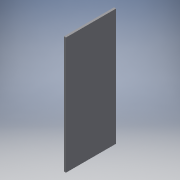
# Autodesk Inventor part: 15102898-16-P-0402
Saved by Autodesk Inventor 2017 (Build 210142000, 142)
## iProperties
Created: 2016-10-08
Part Number: 15102898-16-P-0402
Material: Aluminum 6061
Document SubType Name: Modeling
Designer: gus
Density: 2.7 g/cm^3
Appearance: Aluminum - Flat
Author: gus
Autodesk Inventor part; units mm, degrees
ref_plane "YZ Plane" through (0, 0, 0) normal (1, 0, 0) x (0, 1, 0)
ref_plane "XZ Plane" through (0, 0, 0) normal (0, 1, 0) x (-1, 0, 0)
ref_plane "XY Plane" through (0, 0, 0) normal (0, 0, 1) x (1, 0, 0)
sketch "Sketch1" plane through (0, 0, 0) normal (1, 0, 0) x (0, 1, 0)
  line L0 (0, 0) -> (177.8, 0)
  line L1 (177.8, 0) -> (177.8, -79.375)
  line L2 (177.8, -79.375) -> (0, -79.375)
  line L3 (0, -79.375) -> (0, 0)
  dimension "d0" = 177.8
  dimension "d1" = 79.375
  constraints: 8 end point, 2 parallel, 1 horizontal, 1 perpendicular
  measures "d0" distance of L1.end L2.end
  measures "d1" distance of L0.end L1.end
extrude "Extrusion1" add sketch "Sketch1" along normal blind 3.175
sketch "Sketch2" plane through (3.175, 0, 0) normal (1, 0, 0) x (0, 0, -1)
  line L0 (0, 177.8) -> (0, 0) projected
  line L1 (0, 0) -> (3.175, 0)
  line L2 (3.175, 0) -> (3.175, 177.8)
  line L3 (3.175, 177.8) -> (0, 177.8)
  line L4 (0, 177.8) -> (0, 0)
  dimension "d4" = 3.175
  constraints: 8 end point, 2 parallel, 1 horizontal, 1 perpendicular
  measures "d4" distance between parallel lines of L0 L2
extrude "Extrusion2" add sketch "Sketch2" along normal blind 101.6
sketch "Sketch3" plane through (0, 177.8, 0) normal (0, 1, 0) x (1, 0, 0)
  line L0 (0, 0) -> (104.775, 0) projected
  line L1 (104.775, 0) -> (126.772, -12.7)
  line L2 (126.772, -12.7) -> (128.3595, -9.9504)
  line L3 (128.3595, -9.9504) -> (105.6257, 3.175)
  line L4 (3.175, 3.175) -> (104.775, 3.175) projected
  line L5 (105.6257, 3.175) -> (104.775, 3.175)
  line L6 (3.175, 3.175) -> (104.775, 3.175) projected
  line L7 (104.775, 3.175) -> (104.775, 0) projected
  line L8 (0, 0) -> (104.775, 0) projected
  line L9 (104.775, 3.175) -> (104.775, 0)
  dimension "d7" = 3.175
  dimension "d8" = 25.4
  dimension "d9" = 150
  constraints: 10 end point, 3 perpendicular, 1 collinear
  measures "d7" distance of L1.end L2.end
  measures "d8" distance of L0.end L1.end
  measures "d9" angle of L0 L1
extrude "Extrusion3" add sketch "Sketch3" against normal blind 177.8
body "Solid1"
